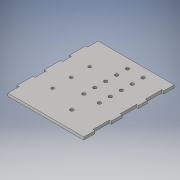
# Autodesk Inventor part: Frontpanel
Saved by Autodesk Inventor 2016 (Build 200138000, 138)
## iProperties
Created: 2016-05-17
Part Number: Frontpanel
Material: Generic
Document SubType Name: Modeling
Designer: Lillahunden
Density: 1 g/cm^3
Appearance: Default
Mass: 190.183 g
Surface Area: 679.872 cm^2
Volume: 190.183 cm^3
Author: Lillahunden
Autodesk Inventor part; units mm, degrees
ref_plane "YZ Plane" through (0, 0, 0) normal (1, 0, 0) x (0, 1, 0)
ref_plane "XZ Plane" through (0, 0, 0) normal (0, 1, 0) x (-1, 0, 0)
ref_plane "XY Plane" through (0, 0, 0) normal (0, 0, 1) x (1, 0, 0)
sketch "Sketch1" plane through (0, 0, 0) normal (0, 0, 1) x (1, 0, 0)
  line L0 (4.1473, 0) -> (4.1473, -28.3717) projected
  line L1 (4.1473, -28.3717) -> (0, -28.3717) projected
  line L2 (0, -6) -> (-159.1383, -6) projected
  line L3 (4.1473, -6) -> (0, -6) projected
  line L4 (0, -28.3717) -> (0, -63.3717) projected
  line L5 (0, -63.3717) -> (4.1473, -63.3717) projected
  line L6 (4.1473, -63.3717) -> (4.1473, -82.5) projected
  line L7 (4.1473, -82.5) -> (0, -82.5) projected
  line L8 (0, -82.5) -> (0, -117.5) projected
  line L9 (4.1473, -117.5) -> (4.1473, -141.25) projected
  line L10 (0, -117.5) -> (4.1473, -117.5) projected
  line L11 (4.1473, -141.25) -> (0, -141.25) projected
  line L12 (0, -141.25) -> (0, -176.25) projected
  line L13 (0, -176.25) -> (4.1473, -176.25) projected
  line L14 (4.1473, -176.25) -> (4.1473, -200) projected
  line L15 (4.1473, -200) -> (0, -200) projected
  line L16 (0, -200) -> (-159.1383, -200) projected
  line L17 (-159.1383, -194) -> (-159.1383, -200) projected
  line L18 (-159.1383, -200) -> (-159.1383, -176.25) projected
  line L19 (-159.1383, -176.25) -> (-163.4742, -176.25) projected
  line L20 (-163.4742, -176.25) -> (-163.4742, -141.25) projected
  line L21 (-163.4742, -141.25) -> (-159.1383, -141.25) projected
  line L22 (-159.1383, -141.25) -> (-159.1383, -117.5) projected
  line L23 (-159.1383, -117.5) -> (-163.4742, -117.5) projected
  line L24 (-163.4742, -117.5) -> (-163.4742, -82.5) projected
  line L25 (-163.4742, -82.5) -> (-159.1383, -82.5) projected
  line L26 (-159.1383, -82.5) -> (-159.1383, -63.3717) projected
  line L27 (-159.1383, -63.3717) -> (-163.4742, -63.3717) projected
  line L28 (-163.4742, -63.3717) -> (-163.4742, -28.3717) projected
  line L29 (-163.4742, -28.3717) -> (-159.1383, -28.3717) projected
  line L30 (-159.1383, -28.3717) -> (-159.1383, 0) projected
  line L31 (-159.1383, -28.3717) -> (-159.1383, 0)
  point P0 (0, 0)
  constraints: 2 end point, 1 vertical, 2 other
extrude "Extrusion1" add sketch "Sketch1" against normal blind 6
sketch "Sketch2" plane through (0, 0, 0) normal (0, 0, 1) x (1, 0, 0)
  circle A0 centre (-75.8527, -120) radius 3.55
  line L0 (-159.1383, -200) -> (4.1473, -200) projected
  line L1 (-163.4742, -141.25) -> (-163.4742, -176.25) projected
  line L2 (4.1473, -200) -> (4.1473, -176.25) projected
  point P0 (0, 0)
  dimension "d2" = 7.1
  dimension "d3" = 80
  dimension "d13" = 80
  constraints: 1 centre point
  measures "d2" diameter of A0
  measures "d3" distance from line of L0 A0.centre
  measures "d13" distance from line of L2 A0.centre
extrude "Extrusion2" cut sketch "Sketch2" against normal through all
pattern_linear "Rectangular Pattern1" count 5 spacing 23.5 along (0, 1, 0) count 2 spacing 33.5 along (1, 0, 0) of "Extrusion2"
sketch "Sketch3" plane through (0, 0, 0) normal (0, 0, 1) x (1, 0, 0)
  circle A0 centre (-42.3527, -120) radius 3.55 construction
  circle A1 centre (-75.8527, -120) radius 3.55 construction
  line L0 (-42.3527, -120) -> (-75.8527, -120) construction
  line L1 (-59.1027, -120) -> (-59.1027, -177.2686) construction
  circle A2 centre (-59.1027, -162.5712) radius 3.6
  point P0 (0, 0)
  dimension "d14" = 7.2
  constraints: 4 end point, 1 centre point, 1 horizontal, 1 midpoint, 1 point on line, 1 vertical
  measures "d14" diameter of A2
extrude "Extrusion3" cut sketch "Sketch3" against normal through all
sketch "Sketch4" plane through (0, 0, 0) normal (0, 0, 1) x (1, 0, 0)
  circle A0 centre (-120.1006, -63) radius 3.1
  line L0 (4.1473, -6) -> (-159.1383, -6) projected
  circle A1 centre (-120.1006, -103) radius 3.1
  circle A2 centre (-120.1006, -143) radius 3.1
  line L1 (-159.1383, -200) -> (4.1473, -200) projected
  point P0 (0, 0)
  dimension "d17" = 6.2
  dimension "d18" = 57
  dimension "d19" = 6.2
  dimension "d20" = 6.2
  dimension "d21" = 40
  dimension "d22" = 40
  dimension "d23" = 57
  constraints: 3 centre point, 2 vertical alignment
  measures "d17" diameter of A0
  measures "d18" distance from line of L0 A0.centre
  measures "d19" diameter of A1
  measures "d20" diameter of A2
  measures "d21" distance of A1.centre A0.centre
  measures "d22" distance of A1.centre A2.centre
  measures "d23" distance from line of L1 A2.centre
extrude "Extrusion4" cut sketch "Sketch4" against normal through all
body "Solid1"
